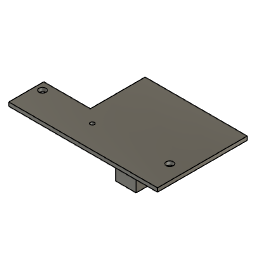
Mainboard_w_supports (Autodesk Fusion 360 archive; units mm, degrees)
design "InputBoard w/ IDC"
Autodesk Fusion 360 part; units mm, degrees
sketch "Sketch1" plane through (0, 0, 0) normal (0, 0, 1) x (1, 0, 0)
  line L0 (0, 0) -> (63.8, 0)
  line L1 (63.8, 0) -> (63.8, 38.5)
  line L2 (63.8, 38.5) -> (0, 38.5)
  line L3 (0, 38.5) -> (0, 0)
  line L4 (0, 15) -> (20, 15)
  line L5 (20, 15) -> (20, 38.5)
  line L6 (63.8, 38.5) -> (43.8, 38.5)
  line L7 (43.8, 38.5) -> (52.6, 38.5)
  line L8 (52.6, 38.5) -> (52.6, 0)
  line L9 (52.6, 0) -> (43.8, 0)
  line L10 (43.8, 0) -> (43.8, 38.5)
  dimension "d1" = 63.8
  dimension "d2" = 38.5
  dimension "d3" = 20
  dimension "d4" = 15
  dimension "d5" = 20
  dimension "d6" = 8.8
  dimension "d7" = 38.5
  constraint horizontal L0
  constraint vertical L1
  constraint horizontal L2
  constraint vertical L3
  constraint coincident L0.start L3.end
  constraint coincident L3 L4.start
  constraint perpendicular L3 L4
  constraint coincident L2 L5.end
  constraint perpendicular L2 L5
  constraint perpendicular L1 L6
  constraint horizontal L7
  constraint vertical L8
  constraint horizontal L9
  constraint vertical L10
  measures "d1" distance of L0.start L0.end
  measures "d2" distance of L0.start L2.end
  measures "d3" distance of L4.start L4.end
  measures "d4" distance of L0 L4
  measures "d5" distance of L1.end L6.end
  measures "d6" distance of L6.end L7.end
  measures "d7" distance of L6.end L9.end
extrude "Extrude2" add sketch "Sketch1" along normal blind 1.6 contours L0 L2 L3 L4 L5 L10 | L0 L2 L6 L7 L8 L9 L10 | L0 L1 L2 L6 L8
sketch "Sketch3" plane through (0, 0, 1.6) normal (0, 0, 1) x (-1, 0, 0)
  line L0 (-63.8, 0) -> (-63.8, -38.5)
  line L1 (-63.8, -38.5) -> (-20, -38.5)
  line L2 (-20, -38.5) -> (-20, -15)
  line L3 (-20, -15) -> (0, -15)
  line L4 (0, -15) -> (0, 0)
  line L5 (0, 0) -> (-63.8, 0)
  line L6 (0, 0) -> (-50, 0) construction
  line L7 (-50, 0) -> (-50, -19.25) construction
  line L8 (-54.4, -0.25) -> (-45.6, -0.25)
  line L9 (-45.6, -0.25) -> (-45.6, -38.25)
  line L10 (-45.6, -38.25) -> (-54.4, -38.25)
  line L11 (-54.4, -38.25) -> (-54.4, -0.25)
  line L12 (-54.4, -0.25) -> (-45.6, -38.25) construction
  line L13 (-45.6, -0.25) -> (-54.4, -38.25) construction
  point P0 (-50, -19.25)
  dimension "d17" = 50
  dimension "d18" = 19.25
  dimension "d19" = 8.8
  dimension "d20" = 38
  constraint coincident L4.end L5.start
  constraint perpendicular L4 L6
  constraint perpendicular L6 L7
  constraint horizontal L8
  constraint perpendicular L8 L9
  constraint parallel L8 L10
  constraint parallel L9 L11
  constraint coincident L12 P0
  constraint coincident L13 P0
  constraint coincident P0 L7.end
  measures "d17" distance of L4.end L6.end
  measures "d18" distance of L6.end P0
  measures "d19" distance of L9.end L10.end
  measures "d20" distance of L8.end L9.end
extrude "Extrude4" add sketch "Sketch3" against normal blind 6.68 contours L8 L9 L10 L11
sketch "Sketch4" plane through (0, 0, 1.6) normal (0, 0, 1) x (-1, 0, 0)
  line L0 (-63.8, 0) -> (-63.8, -38.5)
  line L1 (-63.8, -38.5) -> (-20, -38.5)
  line L2 (-20, -38.5) -> (-20, -15)
  line L3 (-20, -15) -> (0, -15)
  line L4 (0, -15) -> (0, 0)
  line L5 (0, 0) -> (-63.8, 0)
  circle A0 centre (-2.869, -11.6) radius 1.5
  circle A1 centre (-57.479, -11.6) radius 1.5
  dimension "d23" = 3
  dimension "d24" = 11.6
  dimension "d25" = 2.869
  dimension "d28" = 3
  dimension "d29" = 54.61
  dimension "d33" = 57.479
  constraint horizontal A0.centre A1.centre
  measures "d23" diameter of A0
  measures "d24" distance of L5 A0.centre
  measures "d25" distance of L4 A0.centre
  measures "d28" diameter of A1
  measures "d29" distance of A0.centre A1.centre
  measures "d33" distance of L4 A1.centre
extrude "Extrude5" cut sketch "Sketch4" against normal blind 1.6 contours A0
hole "Hole1" at (57.479, 11.6, 1.6) direction (0, 0, -1) diameter 3 depth 5 tip angle 180
sketch "Sketch5" plane through (0, 0, 1.6) normal (0, 0, 1) x (1, 0, 0)
  circle A0 centre (25.907, 9.929) radius 0.85
  line L0 (0, 0) -> (63.8, 0)
  line L1 (0, 15) -> (0, 0)
  dimension "d34" = 1.7
  dimension "d35" = 9.929
  dimension "d36" = 25.907
  measures "d34" diameter of A0
  measures "d35" distance of A0.centre L0
  measures "d36" distance of A0.centre L1
extrude "Extrude6" cut sketch "Sketch5" against normal blind 1.6

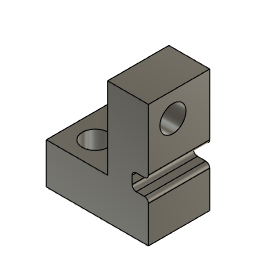
design "Output_Top_Stand"
Autodesk Fusion 360 part; units mm, degrees
sketch "Sketch1" plane through (0, 0, 0) normal (0, 0, 1) x (1, 0, 0)
  line L0 (0, 0) -> (12.5, 0)
  line L1 (12.5, 0) -> (12.5, 7.5)
  line L2 (12.5, 7.5) -> (0, 7.5)
  line L3 (0, 7.5) -> (0, 0)
  dimension "d1" = 12.5
  dimension "d2" = 7.5
  constraint horizontal L0
  constraint vertical L1
  constraint horizontal L2
  constraint vertical L3
  constraint coincident L0.start L3.end
  measures "d1" distance of L0.start L0.end
  measures "d2" distance of L0.start L2.end
extrude "Extrude1" add sketch "Sketch1" along normal blind 5
sketch "Sketch2" plane through (0, 0, 5) normal (0, 0, 1) x (-1, 0, 0)
  line L0 (0, -7.5) -> (0, 0)
  line L1 (0, 0) -> (-12.5, 0)
  line L2 (-12.5, 0) -> (-12.5, -7.5)
  line L3 (-12.5, -7.5) -> (0, -7.5)
  line L4 (-12.5, -7.5) -> (-7.5, -7.5)
  line L5 (-7.5, -7.5) -> (-7.5, 0)
  line L6 (-7.5, 0) -> (-12.5, 0)
  line L7 (-12.5, 0) -> (-12.5, -7.5)
  line L8 (0, -3) -> (-3, -3) construction
  dimension "d5" = 5
  dimension "d6" = 7.5
  dimension "d7" = 3
  dimension "d17" = 3
  constraint horizontal L4
  constraint vertical L5
  constraint horizontal L6
  constraint vertical L7
  constraint coincident L2.end L3.start
  constraint perpendicular L0 L8
  measures "d5" distance of L2.end L4.end
  measures "d6" distance of L2.end L1.end
  measures "d7" distance of L8.start L8.end
  measures "d17" distance of L1 L8
hole "Hole1" at (3, 3, 5) direction (0, 0, -1) diameter 3.2 depth 5 tip angle 180
extrude "Extrude2" add sketch "Sketch2" along normal blind 10 contours L1 L2 L3 L4 L5 L6 L7
sketch "Sketch3" plane through (7.5, 0, 0) normal (-1, 0, 0) x (0, -1, 0)
  line L0 (-7.5, 5) -> (0, 5)
  line L1 (0, 5) -> (0, 15)
  line L2 (0, 15) -> (-7.5, 15)
  line L3 (-7.5, 15) -> (-7.5, 5)
  line L4 (-3, 15) -> (-3, 12) construction
  dimension "d13" = 3
  dimension "d18" = 3
  constraint vertical L4
  measures "d13" distance of L4.start L4.end
  measures "d18" distance of L1 L4
hole "Hole2" at (7.5, 3, 12) direction (1, 0, 0) diameter 3.2 depth 5 tip angle 180
sketch "Sketch4" plane through (12.5, 0, 0) normal (1, 0, 0) x (0, 1, 0)
  circle A0 centre (3, 12) radius 1.6
  line L0 (0, 0) -> (7.5, 0)
  line L1 (7.5, 0) -> (7.5, 15)
  line L2 (7.5, 15) -> (0, 15)
  line L3 (0, 15) -> (0, 0)
  line L4 (0, 6) -> (0, 7)
  line L5 (0, 7) -> (7.5, 7)
  line L6 (7.5, 7) -> (7.5, 5)
  line L7 (7.5, 5) -> (0, 5)
  line L8 (0, 5) -> (0, 7)
  line L9 (0, 0) -> (0, 6)
  dimension "d20" = 1
  dimension "d21" = 2
  dimension "d26" = 6
  constraint coincident L3 L4.start
  constraint horizontal L5
  constraint vertical L6
  constraint horizontal L7
  constraint vertical L8
  constraint midpoint L4.start L8
  constraint coincident L0.start L3.end
  constraint coincident L1 L6.end
  measures "d20" distance of L4.start L4.end
  measures "d21" distance of L4.end L7.end
  measures "d26" distance of L4.start L0.start
extrude "Extrude3" cut sketch "Sketch4" against normal blind 2 contours L1 L3 L4 L5 L6 L7 L8 L9
fillet "Fillet1" radius 0.5 4 edges at (12.5, 3.75, 7) (10.5, 3.75, 7) (10.5, 3.75, 5) (12.5, 3.75, 5)

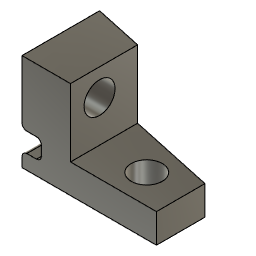
design "Input_Top_Stand"
Autodesk Fusion 360 part; units mm, degrees
sketch "Sketch1" plane through (0, 0, 0) normal (0, 0, 1) x (1, 0, 0)
  line L0 (0, 0) -> (13.866, 0)
  line L1 (13.866, 0) -> (13.866, 5)
  line L2 (0, 4) -> (0, 0)
  line L3 (0, 4) -> (0, 8)
  line L4 (0, 8) -> (13.866, 5)
  dimension "d1" = 13.866
  dimension "d2" = 4
  dimension "d17" = 4
  dimension "d20" = 5
  constraint horizontal L0
  constraint vertical L1
  constraint vertical L2
  constraint coincident L0.start L2.end
  measures "d1" distance of L0.start L0.end
  measures "d2" distance of L0.start L2.start
  measures "d17" distance of L2.start L3.end
  measures "d20" distance of L0.end L1.end
extrude "Extrude1" add sketch "Sketch1" along normal blind 3
sketch "Sketch2" plane through (0, 0, 3) normal (0, 0, 1) x (-1, 0, 0)
  line L0 (0, -8) -> (0, 0)
  line L1 (0, 0) -> (-13.866, 0)
  line L2 (-13.866, 0) -> (-13.866, -5)
  line L3 (-13.866, -3) -> (-9.866, -3) construction
  line L4 (-5, -6.9182) -> (-5, 0)
  line L5 (-5, 0) -> (0, 0)
  line L6 (0, 0) -> (0, -8)
  line L7 (-13.866, -5) -> (0, -8)
  line L8 (0, -8) -> (-5, -6.9182)
  dimension "d5" = 4
  dimension "d7" = 8
  dimension "d19" = 3
  dimension "d21" = 5
  constraint perpendicular L2 L3
  constraint vertical L4
  constraint horizontal L5
  constraint vertical L6
  constraint coincident L0.start L6.end
  constraint coincident L7 L4.start
  measures "d5" distance of L3.start L3.end
  measures "d7" distance of L0.start L0.end
  measures "d19" distance of L1 L3
  measures "d21" distance of L4.end L0.end
hole "Hole1" at (9.866, 3, 3) direction (0, 0, -1) diameter 3.2 depth 5 tip angle 180
extrude "Extrude2" add sketch "Sketch2" along normal blind 7 contours L0 L1 L4 L5 L6 L7 L8
sketch "Sketch3" plane through (5, 0, 0) normal (1, 0, 0) x (0, 1, 0)
  line L0 (0, 3) -> (6.9182, 3)
  line L1 (6.9182, 10) -> (0, 10)
  line L2 (0, 10) -> (0, 3)
  line L3 (3, 10) -> (3, 7.25) construction
  line L4 (6.9182, 3) -> (6.9182, 10)
  dimension "d13" = 2.75
  dimension "d18" = 3
  constraint vertical L3
  constraint coincident L1 L3.start
  measures "d13" distance of L3.start L3.end
  measures "d18" distance of L2 L3
hole "Hole2" at (5, 3, 7.25) direction (-1, 0, 0) diameter 3.2 depth 5 tip angle 180
sketch "Sketch4" plane through (0, 0, 0) normal (-1, 0, 0) x (0, -1, 0)
  line L0 (-8, 0) -> (0, 0)
  line L1 (0, 0) -> (0, 10)
  line L2 (0, 10) -> (-8, 10)
  line L3 (-8, 10) -> (-8, 0)
  line L4 (0, 2.5) -> (0, 3.5)
  line L5 (0, 3.5) -> (-8, 3.5)
  line L6 (-8, 3.5) -> (0, 3.5)
  line L7 (0, 3.5) -> (0, 1.5)
  line L8 (0, 1.5) -> (-8, 1.5)
  line L9 (-8, 1.5) -> (-8, 3.5)
  line L10 (0, 1.5) -> (0, 2.5)
  line L11 (-8, 0.5) -> (-8, 0)
  line L12 (-8, 0) -> (0, 0)
  line L13 (0, 2.5) -> (0, 0)
  circle A0 centre (-3, 7.25) radius 1.6
  dimension "d23" = 1
  dimension "d24" = 2
  dimension "d30" = 2.5
  constraint coincident L1 L4.start
  constraint coincident L3 L5.end
  constraint perpendicular L3 L5
  constraint horizontal L6
  constraint vertical L7
  constraint horizontal L8
  constraint vertical L9
  constraint perpendicular L8 L10
  constraint vertical L11
  constraint horizontal L12
  constraint coincident L0.start L3.end
  constraint perpendicular L12 L13
  measures "d23" distance of L4.start L4.end
  measures "d24" distance of L5.end L8.end
  measures "d30" distance of L4.start L0.end
extrude "Extrude4" cut sketch "Sketch4" against normal blind 2 contours L1 L3 L4 L5 L6 L7 L8 L9 L10 L13
fillet "Fillet2" radius 0.5 4 edges at (2, 3.7836, 1.5) (0, 4, 1.5) (0, 4, 3.5) (2, 3.7836, 3.5)

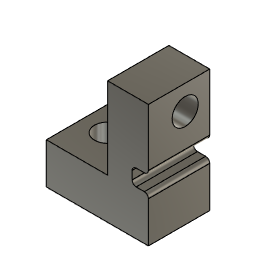
design "Output_Bot_Stand"
Autodesk Fusion 360 part; units mm, degrees
sketch "Sketch1" plane through (0, 0, 0) normal (0, 0, 1) x (1, 0, 0)
  line L0 (0, 0) -> (12.5, 0)
  line L1 (12.5, 0) -> (12.5, 7.5)
  line L2 (12.5, 7.5) -> (0, 7.5)
  line L3 (0, 7.5) -> (0, 0)
  dimension "d1" = 12.5
  dimension "d2" = 7.5
  constraint horizontal L0
  constraint vertical L1
  constraint horizontal L2
  constraint vertical L3
  constraint coincident L0.start L3.end
  measures "d1" distance of L0.start L0.end
  measures "d2" distance of L0.start L2.end
extrude "Extrude1" add sketch "Sketch1" along normal blind 5
sketch "Sketch2" plane through (0, 0, 5) normal (0, 0, 1) x (-1, 0, 0)
  line L0 (0, -7.5) -> (0, 0)
  line L1 (0, 0) -> (-12.5, 0)
  line L2 (-12.5, 0) -> (-12.5, -7.5)
  line L3 (-12.5, -7.5) -> (0, -7.5)
  line L4 (-12.5, -7.5) -> (-7.5, -7.5)
  line L5 (-7.5, -7.5) -> (-7.5, 0)
  line L6 (-7.5, 0) -> (-12.5, 0)
  line L7 (-12.5, 0) -> (-12.5, -7.5)
  line L8 (0, -4.5) -> (-3, -4.5) construction
  dimension "d5" = 5
  dimension "d6" = 7.5
  dimension "d7" = 3
  dimension "d19" = 3
  constraint horizontal L4
  constraint vertical L5
  constraint horizontal L6
  constraint vertical L7
  constraint coincident L2.end L3.start
  constraint perpendicular L0 L8
  measures "d5" distance of L2.end L4.end
  measures "d6" distance of L2.end L1.end
  measures "d7" distance of L8.start L8.end
  measures "d19" distance of L3 L8
hole "Hole1" at (3, 4.5, 5) direction (0, 0, -1) diameter 3.2 depth 5 tip angle 180
extrude "Extrude2" add sketch "Sketch2" along normal blind 10 contours L1 L2 L3 L4 L5 L6 L7
sketch "Sketch3" plane through (7.5, 0, 0) normal (-1, 0, 0) x (0, -1, 0)
  line L0 (-7.5, 5) -> (0, 5)
  line L1 (0, 5) -> (0, 15)
  line L2 (0, 15) -> (-7.5, 15)
  line L3 (-7.5, 15) -> (-7.5, 5)
  line L4 (-4.5, 15) -> (-4.5, 12) construction
  dimension "d13" = 3
  dimension "d20" = 3
  constraint vertical L4
  measures "d13" distance of L4.start L4.end
  measures "d20" distance of L3 L4
hole "Hole2" at (7.5, 4.5, 12) direction (1, 0, 0) diameter 3.2 depth 5 tip angle 180
sketch "Sketch4" plane through (12.5, 0, 0) normal (1, 0, 0) x (0, 1, 0)
  circle A0 centre (4.5, 12) radius 1.6
  line L0 (0, 0) -> (7.5, 0)
  line L1 (7.5, 0) -> (7.5, 15)
  line L2 (7.5, 15) -> (0, 15)
  line L3 (0, 15) -> (0, 0)
  line L4 (4.5, 12) -> (4.5, 7)
  line L5 (4.5, 7) -> (7.5, 7.5)
  line L6 (7.5, 7.5) -> (0, 7.5)
  line L7 (0, 7.5) -> (0, 5.5)
  line L8 (0, 5.5) -> (7.5, 5.5)
  line L9 (7.5, 5.5) -> (7.5, 7.5)
  dimension "d21" = 5
  dimension "d22" = 2
  constraint coincident A0.centre L4.start
  constraint vertical L4
  constraint midpoint L1 L5.end
  constraint horizontal L6
  constraint vertical L7
  constraint horizontal L8
  constraint vertical L9
  constraint coincident L3 L7.end
  measures "d21" distance of A0.centre L4.end
  measures "d22" distance of L5.end L8.end
extrude "Extrude3" cut sketch "Sketch4" against normal blind 2 contours L1 L3 L4 L5 L6 L7 L8 L9 | L4 L5 L6
fillet "Fillet1" radius 0.5 4 edges at (10.5, 3.75, 5.5) (10.5, 3.75, 7.5) (12.5, 3.75, 7.5) (12.5, 3.75, 5.5)

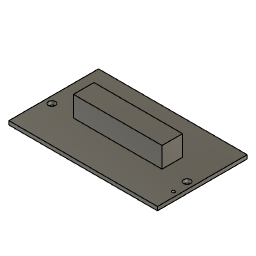
design "Output Board w/ IDC"
Autodesk Fusion 360 part; units mm, degrees
sketch "Sketch1" plane through (0, 0, 0) normal (0, 0, 1) x (1, 0, 0)
  line L0 (0, 0) -> (63.8, 0)
  line L1 (63.8, 0) -> (63.8, 38.5)
  line L2 (63.8, 38.5) -> (0, 38.5)
  line L3 (0, 38.5) -> (0, 0)
  dimension "d1" = 63.8
  dimension "d2" = 38.5
  constraint horizontal L0
  constraint vertical L1
  constraint horizontal L2
  constraint vertical L3
  constraint coincident L0.start L3.end
  measures "d1" distance of L0.start L0.end
  measures "d2" distance of L0.start L2.end
extrude "Extrude1" add sketch "Sketch1" along normal blind 1.6
sketch "Sketch2" plane through (0, 0, 1.6) normal (0, 0, 1) x (-1, 0, 0)
  line L0 (0, -38.5) -> (0, 0)
  line L1 (0, 0) -> (-63.8, 0)
  line L2 (-63.8, 0) -> (-63.8, -38.5)
  line L3 (-63.8, -38.5) -> (0, -38.5)
  line L4 (0, 0) -> (0, -19.25) construction
  line L5 (0, -19.25) -> (-31.9, -19.25) construction
  line L6 (-50.9, -14.85) -> (-12.9, -14.85)
  line L7 (-12.9, -14.85) -> (-12.9, -23.65)
  line L8 (-12.9, -23.65) -> (-50.9, -23.65)
  line L9 (-50.9, -23.65) -> (-50.9, -14.85)
  line L10 (-50.9, -14.85) -> (-12.9, -23.65) construction
  line L11 (-12.9, -14.85) -> (-50.9, -23.65) construction
  point P0 (-31.9, -19.25)
  dimension "d5" = 31.9
  dimension "d6" = 38
  dimension "d7" = 8.8
  constraint coincident L0.end L1.start
  constraint midpoint L0 L4.end
  constraint perpendicular L4 L5
  constraint horizontal L6
  constraint perpendicular L6 L7
  constraint parallel L6 L8
  constraint parallel L7 L9
  constraint coincident L10 P0
  constraint coincident L11 P0
  constraint coincident P0 L5.end
  measures "d5" distance of L4.end P0
  measures "d6" distance of L7.end L8.end
  measures "d7" distance of L6.end L7.end
extrude "Extrude2" add sketch "Sketch2" along normal blind 8.8 contours L6 L7 L8 L9
sketch "Sketch3" plane through (0, 0, 1.6) normal (0, 0, 1) x (-1, 0, 0)
  line L0 (-50.9, -23.65) -> (-50.9, -14.85)
  line L1 (-50.9, -14.85) -> (-12.9, -14.85)
  line L2 (-12.9, -14.85) -> (-12.9, -23.65)
  line L3 (-12.9, -23.65) -> (-50.9, -23.65)
  line L4 (0, -38.5) -> (0, 0)
  line L5 (0, 0) -> (-63.8, 0)
  line L6 (-63.8, 0) -> (-63.8, -38.5)
  line L7 (-63.8, -38.5) -> (0, -38.5)
  circle A0 centre (-60.9, -15.6) radius 1.5
  circle A1 centre (-2.9, -15.6) radius 1.5
  dimension "d10" = 3
  dimension "d11" = 2.9
  dimension "d12" = 15.6
  dimension "d13" = 3
  dimension "d19" = 11.6
  dimension "d21" = 60.9
  dimension "d22" = 2.9
  constraint horizontal A0.centre A1.centre
  measures "d10" diameter of A0
  measures "d11" distance of L6 A0.centre
  measures "d12" distance of L5 A0.centre
  measures "d13" diameter of A1
  measures "d21" distance of L4 A0.centre
  measures "d22" distance of L4 A1.centre
extrude "Extrude4" cut sketch "Sketch3" against normal blind 1.6 contours A0 | A1
sketch "Sketch5" plane through (0, 0, 1.6) normal (0, 0, 1) x (-1, 0, 0)
  circle A0 centre (-2.9, -15.6) radius 1.5
  circle A1 centre (-60.9, -15.6) radius 1.5
  line L0 (-50.9, -23.65) -> (-50.9, -14.85)
  line L1 (-50.9, -14.85) -> (-12.9, -14.85)
  line L2 (-12.9, -14.85) -> (-12.9, -23.65)
  line L3 (-12.9, -23.65) -> (-50.9, -23.65)
  line L4 (0, -38.5) -> (0, 0)
  line L5 (0, 0) -> (-63.8, 0)
  line L6 (-63.8, 0) -> (-63.8, -38.5)
  line L7 (-63.8, -38.5) -> (0, -38.5)
  circle A2 centre (-61.7, -9) radius 0.655
  dimension "d23" = 1.31
  dimension "d28" = 2.1
  dimension "d29" = 9
  measures "d23" diameter of A2
  measures "d28" distance of L6 A2.centre
  measures "d29" distance of L5 A2.centre
extrude "Extrude5" cut sketch "Sketch5" against normal blind 1.6 contours A2

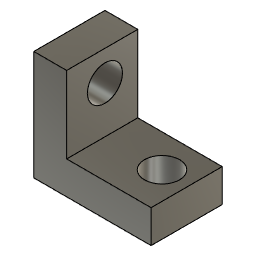
design "Input_Bot_Stand"
Autodesk Fusion 360 part; units mm, degrees
sketch "Sketch1" plane through (0, 0, 0) normal (0, 0, 1) x (1, 0, 0)
  line L0 (0, 0) -> (10.715, 0)
  line L1 (10.715, 0) -> (10.715, 6.5)
  line L2 (10.715, 6.5) -> (0, 6.5)
  line L3 (0, 6.5) -> (0, 0)
  dimension "d1" = 10.715
  dimension "d2" = 6.5
  constraint horizontal L0
  constraint vertical L1
  constraint horizontal L2
  constraint vertical L3
  constraint coincident L0.start L3.end
  measures "d1" distance of L0.start L0.end
  measures "d2" distance of L0.start L2.end
extrude "Extrude1" add sketch "Sketch1" along normal blind 3
sketch "Sketch2" plane through (0, 0, 3) normal (0, 0, 1) x (-1, 0, 0)
  line L0 (0, -6.5) -> (0, 0)
  line L1 (0, 0) -> (-10.715, 0)
  line L2 (-10.715, 0) -> (-10.715, -6.5)
  line L3 (-10.715, -6.5) -> (0, -6.5)
  line L4 (0, -6.5) -> (-3, -6.5)
  line L5 (-3, -6.5) -> (-3, 0)
  line L6 (-3, 0) -> (0, 0)
  line L7 (0, 0) -> (0, -6.5)
  line L8 (-10.715, -3.5) -> (-8.215, -3.5) construction
  dimension "d5" = 3
  dimension "d6" = 6.5
  dimension "d7" = 2.5
  dimension "d17" = 3
  constraint horizontal L4
  constraint vertical L5
  constraint horizontal L6
  constraint vertical L7
  constraint coincident L0.start L3.end
  constraint perpendicular L2 L8
  measures "d5" distance of L0.start L4.end
  measures "d6" distance of L0.start L0.end
  measures "d7" distance of L8.start L8.end
  measures "d17" distance of L3 L8
hole "Hole1" at (8.215, 3.5, 3) direction (0, 0, -1) diameter 3.2 depth 5 tip angle 180
extrude "Extrude2" add sketch "Sketch2" along normal blind 7 contours L0 L1 L3 L4 L5 L6 L7
sketch "Sketch3" plane through (3, 0, 0) normal (1, 0, 0) x (0, 1, 0)
  line L0 (6.5, 10) -> (0, 10)
  line L1 (0, 10) -> (0, 3)
  line L2 (3.5, 10) -> (3.5, 7.25) construction
  line L3 (6.5, 10) -> (3.5, 10)
  line L4 (0, 3) -> (6.5, 3)
  line L5 (6.5, 3) -> (6.5, 10)
  dimension "d13" = 2.75
  dimension "d27" = 3
  constraint perpendicular L0 L2
  constraint coincident L0 L2.start
  constraint coincident L0.start L3.start
  constraint perpendicular L2 L3
  measures "d13" distance of L2.start L2.end
  measures "d27" distance of L2.start L0.start
hole "Hole2" at (3, 3.5, 7.25) direction (-1, 0, 0) diameter 3.2 depth 5 tip angle 180
